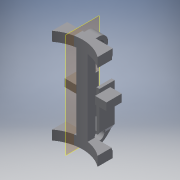
# Autodesk Inventor part: back_pack_3.1
Saved by Autodesk Inventor 2016 (Build 200138000, 138)
## iProperties
Created: 2016-06-06
Part Number: back_pack_3.1
Material: Generic
Document SubType Name: Modeling
Designer: ajar021
Density: 1 g/cm^3
Appearance: Default
Author: ajar021
Autodesk Inventor part; units mm, degrees
ref_plane "YZ Plane" through (0, 0, 0) normal (1, 0, 0) x (0, 1, 0)
ref_plane "XZ Plane" through (0, 0, 0) normal (0, 1, 0) x (-1, 0, 0)
sketch "Sketch1" plane through (0, 0, 0) normal (0, 0, 1) x (1, 0, 0)
  line L0 (-6, 1) -> (6, 1)
  line L1 (6, 1) -> (6, -1)
  line L2 (6, -1) -> (-6, -1)
  line L3 (-6, -1) -> (-6, 1)
  line L4 (-6, 1) -> (6, -1) construction
  line L5 (6, 1) -> (-6, -1) construction
  line L6 (-6, -1) -> (-6, -3)
  line L7 (6, -1) -> (6, -3)
  arc A0 (6, -3) -> (-6, -3) centre (0, -11) ccw
  point P0 (0, 0)
  dimension "d0" = 12
  dimension "d1" = 2
  dimension "d2" = 2
  dimension "d3" = 2
  constraints: 16 end point, 2 midpoint, 2 parallel, 2 point on circle, 2 vertical, 1 centre point, 1 horizontal, 1 perpendicular
  measures "d0" distance of L0.start L0.end
  measures "d1" distance of L0.end L1.end
  measures "d2" distance of L2.end L6.end
  measures "d3" distance of L1.end L7.end
extrude "Extrusion1" add sketch "Sketch1" against normal blind 25
sketch "Sketch2" plane through (-6, 1, 0) normal (0, 1, 0) x (1, 0, 0)
  line L0 (12, 0) -> (12, 25) projected
  line L1 (0, 0) -> (0, 25) projected
  line L2 (0, 0) -> (0, 2.5)
  line L3 (12, 0) -> (12, 2.5)
  line L4 (0, 25) -> (0, 22.5)
  line L5 (12, 25) -> (12, 22.5)
  line L6 (0, 2.5) -> (4.5, 2.5)
  line L7 (4.5, 2.5) -> (4.5, 22.5)
  line L8 (4.5, 22.5) -> (0, 22.5)
  line L9 (0, 22.5) -> (0, 2.5)
  line L10 (12, 2.5) -> (7.5, 2.5)
  line L11 (7.5, 2.5) -> (7.5, 22.5)
  line L12 (7.5, 22.5) -> (12, 22.5)
  line L13 (12, 22.5) -> (12, 2.5)
  point P0 (6, 0)
  dimension "d6" = 2.5
  dimension "d7" = 2.5
  dimension "d8" = 2.5
  dimension "d9" = 2.5
  dimension "d10" = 12
  dimension "d11" = 4.5
  dimension "d12" = 4.5
  constraints: 24 end point, 4 parallel, 4 point on line, 2 horizontal, 2 perpendicular
  measures "d6" distance of L1.start L2.end
  measures "d7" distance of L1.end L4.end
  measures "d8" distance of L0.end L5.end
  measures "d9" distance of L0.start L3.end
  measures "d10" distance of L0.start L1.start
  measures "d11" distance of L8.end L7.end
  measures "d12" distance of L11.end L12.end
extrude "Extrusion2" cut sketch "Sketch2" against normal blind 25
sketch "Sketch3" plane through (-6, 1, 0) normal (0, 1, 0) x (1, 0, 0)
  line L0 (7.5, 2.5) -> (7.5, 22.5) projected
  line L1 (4.5, 22.5) -> (4.5, 2.5) projected
  line L2 (0, 0) -> (0, 2.5) projected
  line L3 (4.5, 2.5) -> (4.5, 3.5)
  line L4 (7.5, 2.5) -> (7.5, 3.5)
  line L5 (4.5, 3.5) -> (4.5, 5)
  line L6 (4.5, 5) -> (5, 5)
  line L7 (5, 5) -> (5, 3.5)
  line L8 (5, 3.5) -> (4.5, 3.5)
  line L9 (7.5, 3.5) -> (7.5, 5)
  line L10 (7.5, 5) -> (7, 5)
  line L11 (7, 5) -> (7, 3.5)
  line L12 (7, 3.5) -> (7.5, 3.5)
  line L13 (4.5, 2.5) -> (4.5, 7)
  line L14 (4.5, 7) -> (0, 7)
  line L15 (0, 7) -> (0, 8.5)
  line L16 (0, 8.5) -> (4.5, 8.5)
  line L17 (7.5, 7) -> (12, 7)
  line L18 (12, 7) -> (12, 8.5)
  line L19 (12, 8.5) -> (7.5, 8.5)
  line L20 (4.5, 7) -> (4.5, 21)
  line L21 (7.5, 7) -> (7.5, 21)
  line L22 (4.5, 21) -> (7.5, 21)
  line L23 (7.5, 21) -> (7.5, 22.5)
  line L24 (7.5, 22.5) -> (4.5, 22.5)
  line L25 (4.5, 22.5) -> (4.5, 21)
  line L26 (4.5, 21) -> (3.5, 21)
  line L27 (3.5, 21) -> (3.5, 11)
  line L28 (3.5, 11) -> (4.5, 11)
  line L29 (4.5, 11) -> (4.5, 21)
  line L30 (7.5, 21) -> (8.5, 21)
  line L31 (8.5, 21) -> (8.5, 11)
  line L32 (8.5, 11) -> (7.5, 11)
  line L33 (7.5, 11) -> (7.5, 21)
  line L34 (3.5, 21) -> (4.5, 22.5)
  line L35 (7.5, 22.5) -> (8.5, 21)
  line L36 (7.5, 5) -> (8, 5)
  line L37 (8, 5) -> (8, 3.5)
  line L38 (8, 3.5) -> (7.5, 3.5)
  line L39 (4.5, 5) -> (4, 5)
  line L40 (4, 5) -> (4, 3.5)
  line L41 (4, 3.5) -> (5, 3.5)
  point P0 (12, 25)
  point P1 (12, 0)
  point P2 (6, 0)
  dimension "d15" = 1
  dimension "d16" = 1.5
  dimension "d17" = 0.5
  dimension "d18" = 0.5
  dimension "d19" = 4.5
  dimension "d20" = 1.5
  dimension "d21" = 14
  dimension "d22" = 4.5
  dimension "d23" = 4.5
  dimension "d24" = 14
  dimension "d25" = 25
  dimension "d26" = 1.5
  dimension "d29" = 1
  dimension "d30" = 10
  dimension "d31" = 1
  dimension "d34" = 0.5
  dimension "d35" = 0.5
  dimension "d50" = 10
  constraints: 78 end point, 20 point on line, 15 perpendicular, 7 parallel, 3 horizontal, 1 collinear
  measures "d15" distance of L1.end L3.end
  measures "d16" distance of L3.end L5.end
  measures "d17" distance of L5.end L6.end
  measures "d18" distance of L9.end L10.end
  measures "d19" distance of L1.end L13.end
  measures "d20" distance of L14.end L15.end
  measures "d21" distance of L13.end L20.end
  measures "d22" distance of L18.end L19.end
  measures "d23" distance of L15.end L16.end
  measures "d24" distance from line of L21.end L17
  measures "d25" distance of point (12, 25) point (12, 0)
  measures "d26" distance of L22.end L23.end
  measures "d29" distance of L28.end L27.end
  measures "d30" distance of L26.end L27.end
  measures "d31" distance of L31.end L32.end
  measures "d34" distance of L9.end L36.end
  measures "d35" distance of L5.end L39.end
  measures "d50" distance of L30.end L31.end
extrude "Extrusion3" add sketch "Sketch3" along normal blind 4 contours L0 L30 L31 L32 | L22 L1 L24 L0 | L0 L35 L30 | L26 L34 L1 | L1 L28 L27 L26
ref_plane "Work Plane1" through (-1.5, 1, -12.5) normal (-1, 0, 0) x (0, 0, 1)
sketch "Sketch8" plane through (-2.5, -1.3175, -11) normal (-1, 0, 0) x (0, 0, 1)
  line L0 (-10, 0) -> (0, 6.3175)
  line L1 (-10, 6.3175) -> (-11.5, 6.3175) projected
  line L2 (0, 0) -> (-10, 0) projected
  line L3 (-10, 6.3175) -> (0, 0)
  line L4 (-4, 1.1588) -> (-4, 5.1588)
  line L5 (-6, 1.1588) -> (-4, 5.1588) construction
  line L6 (-4, 1.1588) -> (-6, 5.1588) construction
  line L7 (-5, 3.1588) -> (-2, 3.1588)
  line L8 (-3, 5.1588) -> (-1, 5.1588)
  line L9 (-1, 5.1588) -> (-1, 1.1588)
  line L10 (-1, 1.1588) -> (-3, 1.1588)
  line L11 (-3, 1.1588) -> (-3, 5.1588)
  line L12 (-3, 5.1588) -> (-1, 1.1588) construction
  line L13 (-1, 5.1588) -> (-3, 1.1588) construction
  line L14 (0, 2.3175) -> (0, 6.3175) projected
  line L15 (-10, 6.3175) -> (0, 6.3175) projected
  line L16 (-6, 5.1588) -> (-3, 5.1588)
  point P0 (11, 1.3175)
  dimension "d51" = 2
  dimension "d52" = 4
  dimension "d103" = 3
  dimension "d104" = 2
  dimension "d105" = 4
  constraints: 26 end point, 5 midpoint, 5 parallel, 3 horizontal, 1 perpendicular
  measures "d51" distance of L6.end L4.end
  measures "d52" distance of L4.start L4.end
  measures "d103" distance of L7.start L7.end
  measures "d104" distance of L9.end L10.end
  measures "d105" distance of L8.end L9.end
extrude "Extrusion8" add sketch "Sketch8" along normal blind 3 contours L10 L11 L3 | L3 L11 L0 L8 L9 L10 | L11 L8 L0
sketch "Sketch9" plane through (2.5, -1.3175, -21) normal (1, 0, 0) x (0, 0, -1)
  line L0 (-10, 6.3175) -> (0, 0)
  line L1 (0, 2.3175) -> (0, 6.3175) projected
  line L2 (0, 0) -> (-10, 0) projected
  line L3 (0, 6.3175) -> (-10, 0)
  line L4 (-6, 5.1588) -> (-6, 1.1588)
  line L5 (-4, 5.1588) -> (-6, 1.1588) construction
  line L6 (-6, 5.1588) -> (-4, 1.1588) construction
  line L7 (-5, 3.1588) -> (-8, 3.1588)
  line L8 (-9, 2.3175) -> (-9, 1.1588) projected
  line L9 (-7, 5.1588) -> (-9, 5.1588)
  line L10 (-9, 5.1588) -> (-9, 1.1588)
  line L11 (-9, 1.1588) -> (-7, 1.1588)
  line L12 (-7, 1.1588) -> (-7, 5.1588)
  line L13 (-7, 5.1588) -> (-9, 1.1588) construction
  line L14 (-9, 5.1588) -> (-7, 1.1588) construction
  point P0 (-21, 1.3175)
  dimension "d55" = 2
  dimension "d56" = 4
  dimension "d106" = 3
  constraints: 24 end point, 7 midpoint, 2 horizontal, 2 parallel, 1 perpendicular
  measures "d55" distance of L6.end L4.end
  measures "d56" distance of L4.end L4.start
  measures "d106" distance of L7.start L7.end
extrude "Extrusion9" add sketch "Sketch9" along normal blind 3 contours L12 L3 L11 L8 L10 L9 L0 | L0 L9 L12 | L12 L11 L3
ref_plane "Work Plane2" through (-2, 1, -11) normal (1, 0, 0) x (0, 0, -1)
sketch "Sketch12" plane through (-2, 1, -11) normal (1, 0, 0) x (0, 0, -1)
  line L0 (11.5, 0) -> (11.5, 4) projected
  line L1 (14, -4) -> (14, 0) projected
  line L2 (14, 0) -> (11.5, 4)
  line L3 (11.5, 0) -> (14, 0) projected
  line L4 (14, 0) -> (11.5, 0)
  line L5 (11.5, 4) -> (12.8115, 3.0819) construction
  line L6 (12.8115, 3.0819) -> (14.0937, 1.3588) construction
  line L7 (14.0937, 1.3588) -> (14, 0) construction
  spline S0 degree 3 poles (11.5, 4) (12.8115, 3.0819) (14.0937, 1.3588) (14, 0) knots 1 1 1 1 2 2 2 2
  point P0 (-11, -1)
  constraints: 4 end point, 1 collinear, 3 other
extrude "Extrusion12" add sketch "Sketch12" along normal up to surface (3.5 mm away)
sketch "Sketch15" plane through (2.5, -1.3175, -21) normal (1, 0, 0) x (0, 0, -1)
  line L0 (1.5, 2.3175) -> (4, 2.3175) projected
  line L1 (1.5, 2.3175) -> (1.5, 6.3175) projected
  line L2 (4, 2.3175) -> (1.5, 2.3175) projected
  line L3 (1.5, 2.3175) -> (1.5, 3.3175)
  circle A0 centre (1.5, 3.3175) radius 1.3
  point P0 (-21, 1.3175)
  dimension "d77" = 1
  dimension "d78" = 2.6
  constraints: 2 end point, 1 centre point, 1 coincident, 1 point on line, 1 other
  measures "d77" distance of L3.start L3.end
  measures "d78" diameter of A0
extrude "Extrusion14" cut sketch "Sketch15" against normal up to surface (12 mm away) from surface at 3.5
sketch "Sketch16" plane through (-6, 5, 0) normal (0, 1, 0) x (1, 0, 0)
  line L0 (3.5, 11) -> (4.5, 11) projected
  line L1 (4.5, 11) -> (4.5, 21) projected
  line L2 (7.5, 21) -> (7.5, 11) projected
  line L3 (7.5, 11) -> (8.5, 11) projected
  line L4 (4.5, 11) -> (4.3, 11)
  line L5 (4.3, 11) -> (4.3, 21)
  line L6 (4.3, 21) -> (4.5, 21)
  line L7 (7.5, 11) -> (7.5, 21) projected
  line L8 (7.5, 11) -> (7.7, 11)
  line L9 (7.7, 11) -> (7.7, 21)
  line L10 (7.7, 21) -> (7.5, 21)
  line L11 (7.5, 21) -> (7.5, 11)
  point P0 (6, 0)
  dimension "d81" = 0.2
  dimension "d82" = 0.2
  dimension "d83" = 0.2
  constraints: 14 end point, 2 equal length, 2 perpendicular, 2 point on line
  measures "d81" distance of L0.end L4.end
  measures "d82" distance of L5.end L1.end
  measures "d83" distance of L2.end L8.end
extrude "Extrusion15" cut sketch "Sketch16" against normal up to surface (4 mm away)
sketch "Sketch17" plane through (1.5, -1.1131, -2.5) normal (1, 0, 0) x (0, 0, -1)
  line L0 (0, 2.1131) -> (18.5, 2.1131) projected
  line L1 (-2.5, 2.1131) -> (0, 2.1131) projected
  line L2 (-2.5, 2.1131) -> (-2.5, 3.1131)
  line L3 (-2.5, 3.1131) -> (-1.5, 3.1131)
  line L4 (-1.5, 3.1131) -> (1, 3.1131)
  line L5 (1, 3.1131) -> (2, 3.1131)
  line L6 (-0.25, 3.1131) -> (-0.25, 4.3631)
  line L7 (-0.25, 4.3631) -> (-0.25, 5.3631)
  line L8 (-2.5, 2.1131) -> (2, 2.1131)
  line L9 (2, 3.1131) -> (2, 2.1131)
  arc A0 (2, 3.1131) -> (-2.5, 3.1131) centre (-0.25, 3.1131) ccw
  dimension "d94" = 1
  dimension "d95" = 1
  dimension "d96" = 2.5
  dimension "d97" = 1
  dimension "d98" = 1.25
  dimension "d99" = 1
  constraints: 16 end point, 3 point on circle, 3 point on line, 3 vertical, 2 perpendicular, 1 centre point, 1 midpoint
  measures "d94" distance of L1.start L2.end
  measures "d95" distance of L2.end L3.end
  measures "d96" distance of L3.end L4.end
  measures "d97" distance of L4.end L5.end
  measures "d98" distance of L6.start L6.end
  measures "d99" distance of L6.end L7.end
extrude "Extrusion16" add sketch "Sketch17" against normal up to surface (3 mm away)
sketch "Sketch19" plane through (6, -3, 0) normal (1, 0, 0) x (0, 0, -1)
  arc A0 (4.5, 5) -> (0, 5) centre (2.25, 5) ccw projected
  circle A1 centre (2.25, 5) radius 1.25
  point P0 (0, 3)
  dimension "d100" = 2.5
  constraints: 1 centre point, 1 coincident
  measures "d100" diameter of A1
extrude "Extrusion17" cut sketch "Sketch19" against normal up to surface (12 mm away)
equation "\"d7\" = d6"
equation "\"d8\" = d6"
equation "\"d9\" = d6"
equation "\"d12\" = d11"
equation "\"d18\" = d17"
equation "\"d22\" = d23"
equation "\"d24\" = d21"
equation "\"d31\" = d29"
equation "\"d50\" = d30"
equation "\"d82\" = d81"
body "Solid1"
